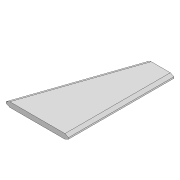
# Autodesk Inventor part: Foam_wing_V2
Saved by Autodesk Inventor 2022 (Build 260153000, 153)
## iProperties
Created: 2022-06-29
Part Number: Foam_wing_V2
Material: Generic
Document SubType Name: Modeling
Designer: dell
Density: 1 g/cm^3
Appearance: Default
Author: dell
Autodesk Inventor part; units mm, degrees
ref_plane "YZ Plane" through (0, 0, 0) normal (1, 0, 0) x (0, 1, 0)
ref_plane "XZ Plane" through (0, 0, 0) normal (0, 1, 0) x (-1, 0, 0)
ref_plane "XY Plane" through (0, 0, 0) normal (0, 0, 1) x (1, 0, 0)
sketch "Sketch1" plane through (0, 0, 0) normal (0, 1, 0) x (-1, 0, 0)
  line L0 (0, 0) -> (355, 0)
  line L1 (355, 0) -> (355, -600)
  line L2 (355, -600) -> (0, -600)
  line L3 (0, -600) -> (0, 0)
  dimension "d0" = 600
  dimension "d1" = 355
  constraints: 8 end point, 2 parallel, 1 horizontal, 1 perpendicular
  measures "d0" distance of L2.end L0.start
  measures "d1" distance of L0.start L0.end
extrude "Extrusion1" add sketch "Sketch1" along normal blind 28
sketch "Sketch2" plane through (0, 28, 0) normal (0, 1, 0) x (1, 0, 0)
  line L0 (-355, 600) -> (-355, 0) projected
  line L1 (0, 600) -> (-355, 600) projected
  line L2 (0, 600) -> (-355, 600) projected
  line L3 (-355, 600) -> (-355, 0) projected
  line L4 (-355, 0) -> (0, 0) projected
  line L5 (0, 0) -> (0, 600) projected
  line L6 (-355, 0) -> (-150, 600)
  point P0 (-150, 600)
  dimension "d7" = 150
  dimension "d8" = 0
  constraints: 2 end point, 2 point on line
  measures "d7" distance of L1.start L6.end
  measures "d8" distance of L0.end L6.start
extrude "Extrusion2" cut sketch "Sketch2" against normal blind 200 contours L1 L6 L0
ref_plane "Work Plane1" through (0, 14, 0) normal (0, 1, 0) x (1, 0, 0)
chamfer "Chamfer1" distance 20 distance2 10 1 edges at (0, 28, -300) measured on face at (-0.5, 28, -300)
chamfer "Chamfer2" distance 10 distance2 20 1 edges at (0, 0, -300) measured on face at (0, 0.5, -300)
chamfer "Chamfer3" distance 20 distance2 10 1 edges at (-252.5, 28, -300) measured on face at (-252.0269, 28, -299.8383)
chamfer "Chamfer4" distance 20 distance2 10 1 edges at (-252.5, 0, -300) measured on face at (-252.0269, 0, -299.8383)
body "Solid1"
